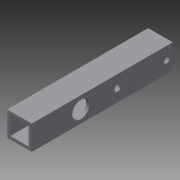
# Autodesk Inventor part: back roller 1x1
Saved by Autodesk Inventor 2015 SP1 (Build 190203100, 203)
## iProperties
Created: 2015-01-25
Part Number: back roller 1x1
Material: Generic
Document SubType Name: Modeling
Designer: Admin
Density: 1 g/cm^3
Appearance: Default
Author: Admin
Autodesk Inventor part; units mm, degrees
ref_plane "YZ Plane" through (0, 0, 0) normal (1, 0, 0) x (0, 1, 0)
ref_plane "XZ Plane" through (0, 0, 0) normal (0, 1, 0) x (-1, 0, 0)
ref_plane "XY Plane" through (0, 0, 0) normal (0, 0, 1) x (1, 0, 0)
sketch "Sketch1" plane through (0, 0, 0) normal (0, 0, 1) x (1, 0, 0)
  line L0 (0, 0) -> (25.4, 0)
  line L1 (25.4, 0) -> (25.4, 25.4)
  line L2 (25.4, 25.4) -> (0, 25.4)
  line L3 (0, 25.4) -> (0, 0)
  line L4 (3.175, 3.175) -> (22.225, 3.175)
  line L5 (22.225, 3.175) -> (22.225, 22.225)
  line L6 (22.225, 22.225) -> (3.175, 22.225)
  line L7 (3.175, 22.225) -> (3.175, 3.175)
  dimension "d0" = 25.4
  dimension "d1" = 25.4
  dimension "d2" = 19.05
  dimension "d3" = 19.05
  dimension "d4" = 3.175
  dimension "d5" = 3.175
  constraints: 16 end point, 4 parallel, 2 horizontal, 2 perpendicular
  measures "d0" distance of L2.end L1.end
  measures "d1" distance of L1.end L0.end
  measures "d2" distance of L6.end L5.end
  measures "d3" distance of L5.end L4.end
  measures "d4" distance between parallel lines of L0 L4
  measures "d5" distance between parallel lines of L3 L7
extrude "Extrusion1" add sketch "Sketch1" along normal blind 146.05
sketch "Sketch2" plane through (0, 0, 0) normal (-1, 0, 0) x (0, 0, 1)
  line L0 (0, 25.4) -> (0, 0) projected
  line L1 (0, 0) -> (146.05, 0) projected
  point P0 (6.35, 12.7)
  point P1 (57.15, 12.7)
  dimension "d8" = 12.7
  dimension "d9" = 6.35
  dimension "d10" = 12.7
  dimension "d11" = 57.15
  measures "d8" distance from line of L1 point (6.35, 12.7)
  measures "d9" distance from line of L0 point (6.35, 12.7)
  measures "d10" distance from line of L1 point (57.15, 12.7)
  measures "d11" distance from line of L0 point (57.15, 12.7)
hole "Hole1" at (0, 12.7, 6.35) at (0, 12.7, 57.15) direction (1, 0, 0) diameter 6.35 end through all
sketch "Sketch3" plane through (25.4, 0, 0) normal (1, 0, 0) x (0, 0, -1)
  line L0 (-146.05, 0) -> (-146.05, 25.4) projected
  line L1 (0, 0) -> (-146.05, 0) projected
  point P0 (-95.25, 12.7)
  dimension "d19" = 50.8
  dimension "d20" = 12.7
  measures "d19" distance from line of L0 point (-95.25, 12.7)
  measures "d20" distance from line of L1 point (-95.25, 12.7)
hole "Hole2" at (25.4, 12.7, 95.25) direction (-1, 0, 0) diameter 17.4625 end through all
body "Solid1"
